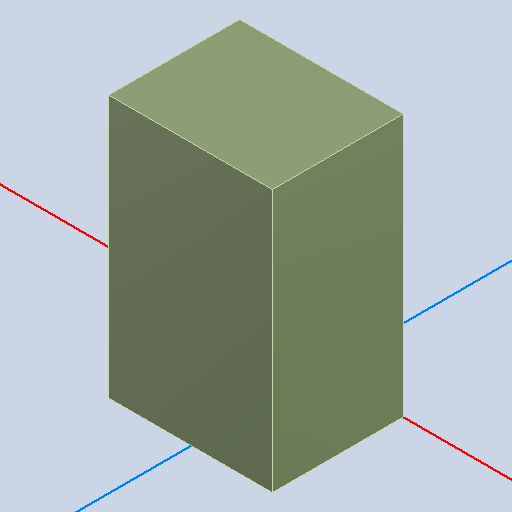
# Autodesk Inventor part: CHIPLED_0805
Saved by Autodesk Inventor 2022 (Build 260153000, 153)
## iProperties
Created: 2022-12-24
Part Number: CHIPLED_0805
Material: Типовые
Document SubType Name: Modeling
Designer: Ivan Petrov
Density: 1 g/cm^3
Appearance: CHIPLED_0805, CHIPLED_0805
Author: Ivan Petrov
Autodesk Inventor part; units mm, degrees
ref_plane "YZ Plane" through (0, 0, 0) normal (1, 0, 0) x (0, 1, 0)
ref_plane "XZ Plane" through (0, 0, 0) normal (0, 1, 0) x (-1, 0, 0)
ref_plane "XY Plane" through (0, 0, 0) normal (0, 0, 1) x (1, 0, 0)
sketch "CHIPLED_0805, CHIPLED_0805_19" plane through (0, 0, 0) normal (0, 0, 1) x (1, 0, 0)
  line L0 (-0.625, 1.0038) -> (0.625, 1.0038)
  line L1 (0.625, 1.0038) -> (0.625, -1)
  line L2 (0.625, -1) -> (-0.625, -1)
  line L3 (-0.625, -1) -> (-0.625, 1.0038)
  constraints: 8 end point
extrude "Выдавливание1" add sketch "CHIPLED_0805, CHIPLED_0805_19" along normal blind 1
